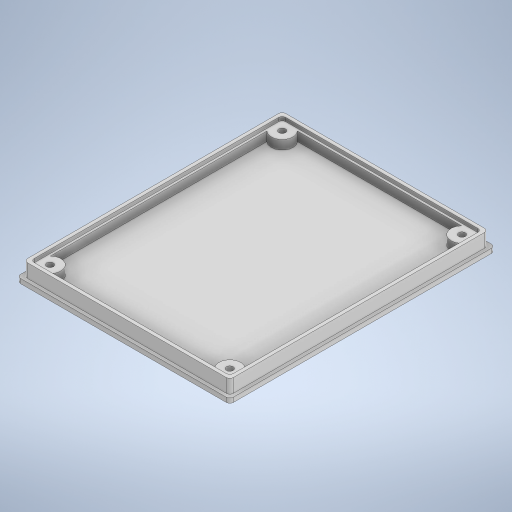
# Autodesk Inventor part: BoardMount
Saved by Autodesk Inventor 2023 (Build 270158000, 158)
## iProperties
Created: 2023-03-22
Part Number: BoardMount
Material: Generic
Document SubType Name: Modeling
Designer: User
Density: 1 g/cm^3
Appearance: Default
Author: User
Autodesk Inventor part; units mm, degrees
ref_plane "YZ Plane" through (0, 0, 0) normal (1, 0, 0) x (0, 1, 0)
ref_plane "XZ Plane" through (0, 0, 0) normal (0, 1, 0) x (-1, 0, 0)
ref_plane "XY Plane" through (0, 0, 0) normal (0, 0, 1) x (1, 0, 0)
sketch "Sketch1" plane through (0, 0, 0) normal (0, 1, 0) x (-1, 0, 0)
  line L0 (-46.75, 58.25) -> (46.75, 58.25)
  line L1 (46.75, 58.25) -> (46.75, -58.25)
  line L2 (46.75, -58.25) -> (-46.75, -58.25)
  line L3 (-46.75, -58.25) -> (-46.75, 58.25)
  line L4 (-46.75, 58.25) -> (46.75, -58.25) construction
  line L5 (46.75, 58.25) -> (-46.75, -58.25) construction
  point P0 (0, 0)
  dimension "d0" = 116.5
  dimension "d1" = 93.5
  constraints: 12 end point, 2 midpoint, 2 parallel, 1 horizontal, 1 perpendicular
  measures "d0" distance of L0.end L1.end
  measures "d1" distance of L1.end L2.end
extrude "Extrusion1" add sketch "Sketch1" along normal blind 8
sketch "Sketch2" plane through (0, 8, 0) normal (0, 1, 0) x (1, 0, 0)
  line L0 (43.75, -55.25) -> (-43.75, -55.25)
  line L1 (-43.75, -55.25) -> (-43.75, 55.25)
  line L2 (-43.75, 55.25) -> (43.75, 55.25)
  line L3 (43.75, 55.25) -> (43.75, -55.25)
  line L4 (43.75, -55.25) -> (-43.75, 55.25) construction
  line L5 (-43.75, -55.25) -> (43.75, 55.25) construction
  point P0 (0, 0)
  dimension "d4" = 110.5
  dimension "d5" = 87.5
  constraints: 12 end point, 2 midpoint, 2 parallel, 1 horizontal, 1 perpendicular
  measures "d4" distance of L0.end L1.end
  measures "d5" distance of L1.end L2.end
extrude "Extrusion2" cut sketch "Sketch2" against normal blind 1.6
sketch "Sketch3" plane through (0, 6.4, 0) normal (0, 1, 0) x (1, 0, 0)
  line L0 (42.75, -54.25) -> (-42.75, -54.25)
  line L1 (-42.75, -54.25) -> (-42.75, 54.25)
  line L2 (-42.75, 54.25) -> (42.75, 54.25)
  line L3 (42.75, 54.25) -> (42.75, -54.25)
  line L4 (42.75, -54.25) -> (-42.75, 54.25) construction
  line L5 (-42.75, -54.25) -> (42.75, 54.25) construction
  point P0 (0, 0)
  dimension "d8" = 108.5
  dimension "d9" = 85.5
  constraints: 12 end point, 2 midpoint, 2 parallel, 1 horizontal, 1 perpendicular
  measures "d8" distance of L0.end L1.end
  measures "d9" distance of L1.end L2.end
extrude "Extrusion3" cut sketch "Sketch3" against normal blind 4
sketch "Sketch4" plane through (0, 2.4, 0) normal (0, 1, 0) x (1, 0, 0)
  circle A0 centre (-39.5, -51) radius 4.75
  circle A1 centre (-39.5, 51) radius 4.75
  line L0 (42.75, -54.25) -> (-42.75, -54.25) projected
  circle A2 centre (39.5, -51) radius 4.75
  line L1 (42.75, 54.25) -> (42.75, -54.25) projected
  circle A3 centre (39.5, 51) radius 4.75
  line L2 (-42.75, -54.25) -> (-42.75, 54.25) projected
  line L3 (-43.75, -55.25) -> (-43.75, 55.25) projected
  line L4 (-43.75, 55.25) -> (43.75, 55.25) projected
  line L5 (43.75, -55.25) -> (-43.75, -55.25) projected
  point P0 (0, 0)
  point P1 (-42.75, 54.25)
  point P2 (-42.75, -47.5359)
  point P3 (-36.0359, -54.25)
  point P4 (42.75, -47.5359)
  point P5 (36.0359, -54.25)
  point P6 (41, 55.25)
  point P7 (41, -55.25)
  point P8 (-41, -55.25)
  point P9 (-41, 55.25)
  dimension "d12" = 9.5
  dimension "d13" = 9.5
  dimension "d14" = 102
  dimension "d17" = 9.5
  dimension "d20" = 79
  dimension "d21" = 9.5
  dimension "d22" = 102
  dimension "d23" = 79
  dimension "d42" = 4.25
  dimension "d43" = 4.25
  dimension "d44" = 4.25
  dimension "d45" = 4.25
  constraints: 4 centre point, 2 other
  measures "d12" diameter of A0
  measures "d13" diameter of A1
  measures "d14" distance of A1.centre A0.centre
  measures "d17" diameter of A2
  measures "d20" distance of A2.centre A0.centre
  measures "d21" diameter of A3
  measures "d22" distance of A3.centre A2.centre
  measures "d23" distance of A3.centre A1.centre
  measures "d42" distance from line of L3 A1.centre
  measures "d43" distance from line of L4 A1.centre
  measures "d44" distance from line of L3 A0.centre
  measures "d45" distance from line of L5 A2.centre
extrude "Extrusion4" add sketch "Sketch4" along normal blind 4 contours A0 L0 L2 | L2 L0 A0 L5 L3 | L3 A0 | A1 L3 L4 | A0 L5 | A2 L1 L0 | L0 L1 A2 L5 | A1 L3 | L5 A2 | L4 A1 | A3 L4 | A3 L4 picked at (-38.9284, 52.0845)
sketch "Sketch5" plane through (0, 6.4, 0) normal (0, 1, 0) x (1, 0, 0)
  arc A0 (-36.0359, -54.25) -> (-42.75, -47.5359) centre (-39.5, -51) ccw projected
  circle A1 centre (-39.5, -51) radius 1.5
  arc A2 (-42.75, 47.5359) -> (-36.0359, 54.25) centre (-39.5, 51) ccw projected
  circle A3 centre (-39.5, 51) radius 1.5
  arc A4 (36.0359, 54.25) -> (42.75, 47.5359) centre (39.5, 51) ccw projected
  circle A5 centre (39.5, 51) radius 1.5
  arc A6 (42.75, -47.5359) -> (36.0359, -54.25) centre (39.5, -51) ccw projected
  circle A7 centre (39.5, -51) radius 1.5
  point P0 (0, 0)
  point P1 (-41.8318, -54.25)
  dimension "d27" = 3
  dimension "d28" = 3
  dimension "d29" = 3
  dimension "d30" = 3
  constraints: 4 centre point, 4 coincident
  measures "d27" diameter of A1
  measures "d28" diameter of A3
  measures "d29" diameter of A5
  measures "d30" diameter of A7
extrude "Extrusion5" cut sketch "Sketch5" against normal blind 4
fillet "Fillet1" radius 1.5 4 edges at (-43.75, 7.2, 55.25) (-43.75, 7.2, -55.25) (43.75, 7.2, 55.25) (43.75, 7.2, -55.25)
sketch "Sketch6" plane through (0, 8, 0) normal (0, 1, 0) x (1, 0, 0)
  line L0 (45.25, -56.75) -> (-45.25, -56.75)
  line L1 (-45.25, -56.75) -> (-45.25, 56.75)
  line L2 (-45.25, 56.75) -> (45.25, 56.75)
  line L3 (45.25, 56.75) -> (45.25, -56.75)
  line L4 (45.25, -56.75) -> (-45.25, 56.75) construction
  line L5 (-45.25, -56.75) -> (45.25, 56.75) construction
  line L6 (50, -69.25) -> (-50, -69.25)
  line L7 (-50, -69.25) -> (-50, 69.25)
  line L8 (-50, 69.25) -> (50, 69.25)
  line L9 (50, 69.25) -> (50, -69.25)
  line L10 (50, -69.25) -> (-50, 69.25) construction
  line L11 (-50, -69.25) -> (50, 69.25) construction
  point P0 (0, 0)
  dimension "d35" = 113.5
  dimension "d36" = 90.5
  dimension "d37" = 138.5
  dimension "d38" = 100
  constraints: 24 end point, 4 midpoint, 4 parallel, 2 horizontal, 2 perpendicular
  measures "d35" distance of L0.end L1.end
  measures "d36" distance of L1.end L2.end
  measures "d37" distance of L6.end L7.end
  measures "d38" distance of L7.end L8.end
extrude "Extrusion6" cut sketch "Sketch6" against normal blind 6
fillet "Fillet3" radius 1.5 8 edges at (45.25, 5, 56.75) (46.75, 1, 58.25) (45.25, 5, -56.75) (46.75, 1, -58.25) (-45.25, 5, -56.75) (-46.75, 1, -58.25) (-45.25, 5, 56.75) (-46.75, 1, 58.25)
body "Solid1"
